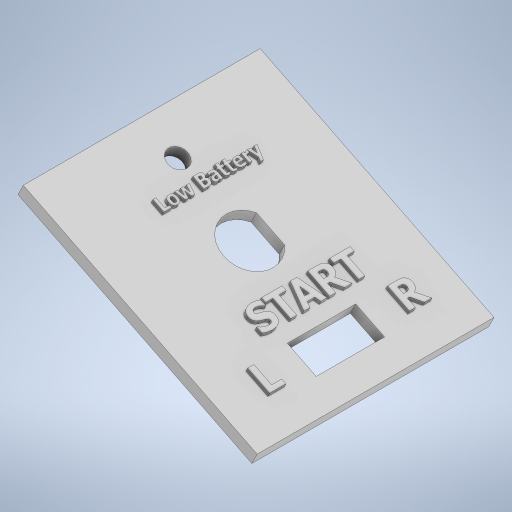
# Autodesk Inventor part: ControlPanel_Top
Saved by Autodesk Inventor 2024.2 (Build 282272000, 272)
## iProperties
Created: 2024-04-16
Part Number: ControlPanel_Top
Material: Generic
Document SubType Name: Modeling
Designer: ringl
Density: 1 g/cm^3
Appearance: Default
Author: ringl
Autodesk Inventor part; units mm, degrees
note: some values were not read from the file. Chosen so that the rebuilt part matches the saved one: direction of "Emboss1".
ref_plane "YZ Plane" through (0, 0, 0) normal (1, 0, 0) x (0, 1, 0)
ref_plane "XZ Plane" through (0, 0, 0) normal (0, 1, 0) x (-1, 0, 0)
ref_plane "XY Plane" through (0, 0, 0) normal (0, 0, 1) x (1, 0, 0)
sketch "Sketch2" plane through (0, 0, 0) normal (0, 0, 1) x (1, 0, 0)
  line L0 (0, 0) -> (1.3327, 2.6877)
  line L1 (1.3327, 2.6877) -> (-36.9173, 21.6547)
  line L2 (-36.9173, 21.6547) -> (-38.25, 18.9669)
  line L3 (-38.25, 18.9669) -> (0, 0)
  line L4 (-38.25, 18.9669) -> (-38.25, 15)
  line L5 (-38.25, 15) -> (-30.25, 15)
  line L6 (-6.5, 3.2231) -> (-6.5, 0)
  line L7 (-6.5, 0) -> (0, 0)
  line L8 (1.3327, 2.6877) -> (21.3327, -7.2296)
  line L9 (21.3327, -7.2296) -> (20, -9.9174)
  line L10 (20, -9.9174) -> (0, 0)
  point P0 (-3.25, 0)
  point P1 (-34.25, 15)
  dimension "d4" = 3
  dimension "d5" = 3
  dimension "d6" = 38.25
  dimension "d8" = 6.5
  dimension "d9" = 8
  dimension "d16" = 15
  dimension "d29" = 20
  constraints: 22 end point, 5 perpendicular, 2 collinear, 2 midpoint, 2 point on line, 2 vertical
  measures "d4" distance of L0.start L0.end
  measures "d5" distance of L1.end L2.end
  measures "d6" horizontal distance of L0.end L1.end
  measures "d8" distance of L6.end L0.start
  measures "d9" distance of L4.end L5.end
  measures "d16" vertical distance of point (-3.25, 0) point (-34.25, 15)
  measures "d29" horizontal distance of L0.end L8.end
extrude "Extrusion1" add sketch "Sketch2" along normal blind 9
sketch "Sketch3" plane through (0, 0, 9) normal (0, 0, 1) x (1, 0, 0)
  line L0 (-38.25, 18.9669) -> (-38.25, 15) projected
  line L1 (-38.25, 15) -> (-30.25, 15) projected
  line L2 (-30.25, 15) -> (-6.5, 3.2231) projected
  line L3 (-6.5, 3.2231) -> (-6.5, 0) projected
  line L4 (-6.5, 0) -> (0, 0) projected
  line L5 (-36.9173, 21.6547) -> (-38.25, 18.9669) projected
  line L6 (-30.25, 15) -> (-38.25, 18.9669)
  line L7 (-6.5, 3.2231) -> (0, 0)
  line L8 (0, 0) -> (20, -9.9174) projected
  line L9 (20, -9.9174) -> (21.3327, -7.2296) projected
  line L10 (21.3327, -7.2296) -> (-36.9173, 21.6547) projected
  constraints: 4 end point
extrude "Extrusion2" add sketch "Sketch3" along normal blind 41 contours L5 L10 L9 L8 L7 L2 L6
sketch "Sketch4" plane through (0, 0, 50) normal (0, 0, 1) x (1, 0, 0)
  line L0 (-38.25, 15) -> (-30.25, 15) projected
  line L1 (-30.25, 15) -> (-38.25, 18.9669) projected
  line L2 (-38.25, 18.9669) -> (-38.25, 15) projected
  line L3 (-38.25, 15) -> (-30.25, 15) projected
  line L4 (-36.9173, 21.6547) -> (-38.25, 18.9669) projected
  line L5 (-38.25, 18.9669) -> (20, -9.9174) projected
  line L6 (0, 0) -> (-6.5, 3.2231) projected
  line L7 (-6.5, 3.2231) -> (-6.5, 0) projected
  line L8 (-6.5, 0) -> (0, 0) projected
  line L9 (20, -9.9174) -> (21.3327, -7.2296) projected
  line L10 (21.3327, -7.2296) -> (-36.9173, 21.6547) projected
  point P0 (-6.5, 3.2231)
extrude "Extrusion3" add sketch "Sketch4" along normal blind 9
sketch "Sketch7" plane through (-36.9173, 21.6547, 59) normal (0.4442495, 0.8959031, 0) x (0.8959031, -0.4442495, 0)
  circle A0 centre (10, 29.5) radius 2.5
  arc A1 (26.1, 34.7) -> (33.9, 34.7) centre (30, 29.5) ccw
  line L0 (50, 21) -> (58, 21)
  line L1 (58, 21) -> (58, 38)
  line L2 (58, 38) -> (50, 38)
  line L3 (50, 38) -> (50, 21)
  line L4 (65.0182, 0) -> (0, 0) projected
  line L5 (26.1, 34.7) -> (33.9, 34.7)
  line L6 (0, 59) -> (0, 0) projected
  point P0 (42.6943, 59)
  point P1 (30, 34.7)
  dimension "d30" = 5
  dimension "d31" = 13
  dimension "d32" = 29.5
  dimension "d33" = 17
  dimension "d34" = 5.2
  dimension "d35" = 10
  dimension "d36" = 20
  dimension "d37" = 8
  dimension "d38" = 8.5
  dimension "d39" = 20
  constraints: 10 end point, 2 centre point, 2 horizontal, 2 parallel, 2 point on circle, 1 horizontal alignment, 1 midpoint, 1 perpendicular
  measures "d30" diameter of A0
  measures "d31" diameter of A1
  measures "d32" distance from line of L4 A0.centre
  measures "d33" distance of L0.end L1.end
  measures "d34" distance of A1.centre point (30, 34.7)
  measures "d35" distance from line of L6 A0.centre
  measures "d36" distance of A0.centre A1.centre
  measures "d37" distance of L1.end L2.end
  measures "d38" distance from line of A1.centre L0
  measures "d39" distance from line of A1.centre L3
extrude "Extrusion5" cut sketch "Sketch7" against normal through all
sketch "Sketch8" plane through (-36.9173, 21.6547, 59) normal (0.4442495, 0.8959031, 0) x (0.8959031, -0.4442495, 0)
  line L0 (50.6129, 9.4648) -> (50.6129, 15.8675) construction
  line L1 (50.6129, 15.8675) -> (57.6973, 15.8675) construction
  line L2 (57.6973, 15.8675) -> (57.6973, 9.4648) construction
  line L3 (57.6973, 9.4648) -> (50.6129, 9.4648) construction
  line L4 (50.3694, 44.5006) -> (50.3694, 50.5681) construction
  line L5 (50.3694, 50.5681) -> (57.1811, 50.5681) construction
  line L6 (57.1811, 50.5681) -> (57.1811, 44.5006) construction
  line L7 (57.1811, 44.5006) -> (50.3694, 44.5006) construction
  line L8 (40.4621, 17.2085) -> (40.4621, 23.6112) construction
  line L9 (40.4621, 23.6112) -> (47.5465, 23.6112) construction
  line L10 (47.5465, 23.6112) -> (47.5465, 17.2085) construction
  line L11 (47.5465, 17.2085) -> (40.4621, 17.2085) construction
  line L12 (19.3245, 18.3628) -> (14.6791, 18.3628) construction
  line L13 (14.6791, 18.3628) -> (14.6791, 42.9569) construction
  line L14 (14.6791, 42.9569) -> (19.3245, 42.9569) construction
  line L15 (19.3245, 42.9569) -> (19.3245, 18.3628) construction
  line L16 (56.7129, 14.1658) -> (56.7129, 10.0975)
  line L17 (56.7129, 10.0975) -> (50.6129, 10.0975)
  line L18 (50.6129, 10.0975) -> (50.6129, 11.6299)
  line L19 (50.6129, 11.6299) -> (55.5512, 11.6299)
  line L20 (55.5512, 11.6299) -> (55.5512, 14.1658)
  line L21 (55.5512, 14.1658) -> (56.7129, 14.1658)
  line L22 (56.4694, 50.7687) -> (56.4694, 48.905)
  line L23 (56.4694, 48.905) -> (54.2301, 47.2095)
  line L24 (54.2301, 47.2095) -> (54.2301, 46.6559)
  line L25 (54.2301, 46.6559) -> (56.4694, 46.6559)
  line L26 (56.4694, 46.6559) -> (56.4694, 45.1333)
  line L27 (56.4694, 45.1333) -> (50.3694, 45.1333)
  line L28 (50.3694, 45.1333) -> (50.3694, 47.5852)
  spline S0 degree 2 poles (50.3694, 47.5852) (50.3694, 48.0943) (50.4979, 48.8457) (50.6956, 49.167) knots 0 0 0 1 2 2 2
  spline S1 degree 2 poles (50.6956, 49.167) (50.9032, 49.4933) (51.5508, 49.8789) (52.0451, 49.8789) knots 0 0 0 1 2 2 2
  spline S2 degree 2 poles (52.0451, 49.8789) (52.7421, 49.8789) (53.6171, 49.2461) (53.8741, 48.7172) knots 0 0 0 1 2 2 2
  line L29 (53.8741, 48.7172) -> (56.4694, 50.7687)
  spline S3 degree 2 poles (52.2379, 48.3069) (52.0056, 48.3069) (51.6744, 48.129) (51.5854, 47.9263) knots 0 0 0 1 2 2 2
  spline S4 degree 2 poles (51.5854, 47.9263) (51.5261, 47.7829) (51.4915, 47.4319) (51.4915, 47.17) knots 0 0 0 1 2 2 2
  line L30 (51.4915, 47.17) -> (51.4915, 46.6559)
  line L31 (51.4915, 46.6559) -> (53.1326, 46.6559)
  line L32 (53.1326, 46.6559) -> (53.1326, 47.0958)
  spline S5 degree 2 poles (53.1326, 47.0958) (53.1326, 47.4122) (53.0536, 47.862) (52.93, 48.0153) knots 0 0 0 1 2 2 2
  spline S6 degree 2 poles (52.93, 48.0153) (52.8113, 48.1636) (52.495, 48.3069) (52.2379, 48.3069) knots 0 0 0 1 2 2 2
  spline S7 degree 2 poles (46.7796, 19.7246) (46.7796, 19.0227) (46.5077, 17.9648) (46.31, 17.51) knots 0 0 0 1 2 2 2
  line L33 (46.31, 17.51) -> (44.8567, 17.51)
  line L34 (44.8567, 17.51) -> (44.8567, 17.6484)
  spline S8 degree 2 poles (44.8567, 17.6484) (45.2472, 18.1081) (45.6674, 19.2105) (45.6674, 19.7295) knots 0 0 0 1 2 2 2
  spline S9 degree 2 poles (45.6674, 19.7295) (45.6674, 19.863) (45.6081, 20.2931) (45.5487, 20.4216) knots 0 0 0 1 2 2 2
  spline S10 degree 2 poles (45.5487, 20.4216) (45.4795, 20.5798) (45.2274, 20.8022) (45.0248, 20.8022) knots 0 0 0 1 2 2 2
  spline S11 degree 2 poles (45.0248, 20.8022) (44.7924, 20.8022) (44.5057, 20.4414) (44.4415, 20.1942) knots 0 0 0 1 2 2 2
  spline S12 degree 2 poles (44.4415, 20.1942) (44.3574, 19.8828) (44.2141, 19.1759) (44.1053, 18.8645) knots 0 0 0 1 2 2 2
  spline S13 degree 2 poles (44.1053, 18.8645) (43.8581, 18.1576) (43.0128, 17.5446) (42.3801, 17.5446) knots 0 0 0 1 2 2 2
  spline S14 degree 2 poles (42.3801, 17.5446) (41.5249, 17.5446) (40.4621, 18.993) (40.4621, 20.0805) knots 0 0 0 1 2 2 2
  spline S15 degree 2 poles (40.4621, 20.0805) (40.4621, 20.6243) (40.6846, 21.7019) (40.8724, 22.127) knots 0 0 0 1 2 2 2
  line L35 (40.8724, 22.127) -> (42.2664, 22.127)
  line L36 (42.2664, 22.127) -> (42.2664, 21.9936)
  spline S16 degree 2 poles (42.2664, 21.9936) (41.9748, 21.6525) (41.5744, 20.6737) (41.5744, 20.1596) knots 0 0 0 1 2 2 2
  spline S17 degree 2 poles (41.5744, 20.1596) (41.5744, 19.9569) (41.6337, 19.6406) (41.7128, 19.4626) knots 0 0 0 1 2 2 2
  spline S18 degree 2 poles (41.7128, 19.4626) (41.777, 19.3193) (42.0341, 19.1116) (42.1923, 19.1116) knots 0 0 0 1 2 2 2
  spline S19 degree 2 poles (42.1923, 19.1116) (42.4295, 19.1116) (42.7014, 19.4428) (42.8102, 19.9174) knots 0 0 0 1 2 2 2
  spline S20 degree 2 poles (42.8102, 19.9174) (42.8794, 20.2239) (43.0128, 20.7923) (43.1265, 21.1186) knots 0 0 0 1 2 2 2
  spline S21 degree 2 poles (43.1265, 21.1186) (43.3589, 21.7513) (44.13, 22.3693) (44.7628, 22.3693) knots 0 0 0 1 2 2 2
  spline S22 degree 2 poles (44.7628, 22.3693) (45.6723, 22.3693) (46.7796, 20.9406) (46.7796, 19.7246) knots 0 0 0 1 2 2 2
  line L37 (46.6709, 24.3268) -> (41.7325, 24.3268)
  line L38 (41.7325, 24.3268) -> (41.7325, 22.5225)
  line L39 (41.7325, 22.5225) -> (40.5709, 22.5225)
  line L40 (40.5709, 22.5225) -> (40.5709, 27.6635)
  line L41 (40.5709, 27.6635) -> (41.7325, 27.6635)
  line L42 (41.7325, 27.6635) -> (41.7325, 25.8592)
  line L43 (41.7325, 25.8592) -> (46.6709, 25.8592)
  line L44 (46.6709, 25.8592) -> (46.6709, 24.3268)
  line L45 (46.6709, 27.6338) -> (40.5709, 29.6952)
  line L46 (40.5709, 29.6952) -> (40.5709, 31.366)
  line L47 (40.5709, 31.366) -> (46.6709, 33.4274)
  line L48 (46.6709, 33.4274) -> (46.6709, 31.8505)
  line L49 (46.6709, 31.8505) -> (45.4252, 31.4698)
  line L50 (45.4252, 31.4698) -> (45.4252, 29.5518)
  line L51 (45.4252, 29.5518) -> (46.6709, 29.1663)
  line L52 (46.6709, 29.1663) -> (46.6709, 27.6338)
  line L53 (44.3179, 31.1337) -> (42.301, 30.5108)
  line L54 (42.301, 30.5108) -> (44.3179, 29.883)
  line L55 (44.3179, 29.883) -> (44.3179, 31.1337)
  line L56 (46.6709, 39.6707) -> (46.6709, 37.8071)
  line L57 (46.6709, 37.8071) -> (44.4316, 36.1116)
  line L58 (44.4316, 36.1116) -> (44.4316, 35.5579)
  line L59 (44.4316, 35.5579) -> (46.6709, 35.5579)
  line L60 (46.6709, 35.5579) -> (46.6709, 34.0354)
  line L61 (46.6709, 34.0354) -> (40.5709, 34.0354)
  line L62 (40.5709, 34.0354) -> (40.5709, 36.4872)
  spline S23 degree 2 poles (40.5709, 36.4872) (40.5709, 36.9964) (40.6994, 37.7478) (40.8971, 38.0691) knots 0 0 0 1 2 2 2
  spline S24 degree 2 poles (40.8971, 38.0691) (41.1047, 38.3953) (41.7523, 38.7809) (42.2466, 38.7809) knots 0 0 0 1 2 2 2
  spline S25 degree 2 poles (42.2466, 38.7809) (42.9436, 38.7809) (43.8186, 38.1482) (44.0757, 37.6193) knots 0 0 0 1 2 2 2
  line L63 (44.0757, 37.6193) -> (46.6709, 39.6707)
  spline S26 degree 2 poles (42.4394, 37.209) (42.2071, 37.209) (41.8759, 37.031) (41.7869, 36.8283) knots 0 0 0 1 2 2 2
  spline S27 degree 2 poles (41.7869, 36.8283) (41.7276, 36.685) (41.693, 36.334) (41.693, 36.072) knots 0 0 0 1 2 2 2
  line L64 (41.693, 36.072) -> (41.693, 35.5579)
  line L65 (41.693, 35.5579) -> (43.3342, 35.5579)
  line L66 (43.3342, 35.5579) -> (43.3342, 35.9979)
  spline S28 degree 2 poles (43.3342, 35.9979) (43.3342, 36.3142) (43.2551, 36.7641) (43.1315, 36.9173) knots 0 0 0 1 2 2 2
  spline S29 degree 2 poles (43.1315, 36.9173) (43.0128, 37.0656) (42.6965, 37.209) (42.4394, 37.209) knots 0 0 0 1 2 2 2
  line L67 (46.6709, 41.297) -> (41.7325, 41.297)
  line L68 (41.7325, 41.297) -> (41.7325, 39.4928)
  line L69 (41.7325, 39.4928) -> (40.5709, 39.4928)
  line L70 (40.5709, 39.4928) -> (40.5709, 44.6338)
  line L71 (40.5709, 44.6338) -> (41.7325, 44.6338)
  line L72 (41.7325, 44.6338) -> (41.7325, 42.8295)
  line L73 (41.7325, 42.8295) -> (46.6709, 42.8295)
  line L74 (46.6709, 42.8295) -> (46.6709, 41.297)
  line L75 (17.7291, 20.7134) -> (17.7291, 18.6792)
  line L76 (17.7291, 18.6792) -> (14.6791, 18.6792)
  line L77 (14.6791, 18.6792) -> (14.6791, 19.4454)
  line L78 (14.6791, 19.4454) -> (17.1483, 19.4454)
  line L79 (17.1483, 19.4454) -> (17.1483, 20.7134)
  line L80 (17.1483, 20.7134) -> (17.7291, 20.7134)
  spline S30 degree 2 poles (16.5798, 23.2443) (17.1483, 23.2443) (17.8008, 22.6239) (17.8008, 22.0579) knots 0 0 0 1 2 2 2
  spline S31 degree 2 poles (17.8008, 22.0579) (17.8008, 21.4944) (17.1483, 20.8691) (16.5798, 20.8691) knots 0 0 0 1 2 2 2
  spline S32 degree 2 poles (16.5798, 20.8691) (16.0064, 20.8691) (15.3563, 21.4944) (15.3563, 22.0579) knots 0 0 0 1 2 2 2
  spline S33 degree 2 poles (15.3563, 22.0579) (15.3563, 22.6215) (16.0088, 23.2443) (16.5798, 23.2443) knots 0 0 0 1 2 2 2
  spline S34 degree 2 poles (16.5847, 22.5102) (16.3796, 22.5102) (16.1052, 22.4435) (16.0237, 22.3842) knots 0 0 0 1 2 2 2
  spline S35 degree 2 poles (16.0237, 22.3842) (15.9372, 22.3199) (15.8704, 22.1593) (15.8704, 22.0579) knots 0 0 0 1 2 2 2
  spline S36 degree 2 poles (15.8704, 22.0579) (15.8704, 21.9591) (15.9298, 21.8033) (16.0138, 21.7391) knots 0 0 0 1 2 2 2
  spline S37 degree 2 poles (16.0138, 21.7391) (16.0929, 21.6773) (16.3722, 21.6031) (16.5847, 21.6031) knots 0 0 0 1 2 2 2
  spline S38 degree 2 poles (16.5847, 21.6031) (16.7948, 21.6031) (17.0543, 21.6724) (17.1334, 21.7292) knots 0 0 0 1 2 2 2
  spline S39 degree 2 poles (17.1334, 21.7292) (17.2125, 21.786) (17.2867, 21.9591) (17.2867, 22.0629) knots 0 0 0 1 2 2 2
  spline S40 degree 2 poles (17.2867, 22.0629) (17.2867, 22.1494) (17.2125, 22.3273) (17.1384, 22.3817) knots 0 0 0 1 2 2 2
  spline S41 degree 2 poles (17.1384, 22.3817) (17.0519, 22.4435) (16.8022, 22.5102) (16.5847, 22.5102) knots 0 0 0 1 2 2 2
  line L81 (15.428, 27.0531) -> (17.7291, 26.3808)
  line L82 (17.7291, 26.3808) -> (17.7291, 25.6196)
  line L83 (17.7291, 25.6196) -> (16.2412, 25.2142)
  line L84 (16.2412, 25.2142) -> (17.7291, 24.8089)
  line L85 (17.7291, 24.8089) -> (17.7291, 24.0476)
  line L86 (17.7291, 24.0476) -> (15.428, 23.3803)
  line L87 (15.428, 23.3803) -> (15.428, 24.1341)
  line L88 (15.428, 24.1341) -> (16.9505, 24.4875)
  line L89 (16.9505, 24.4875) -> (15.428, 24.9226)
  line L90 (15.428, 24.9226) -> (15.428, 25.5578)
  line L91 (15.428, 25.5578) -> (16.9505, 25.9681)
  line L92 (16.9505, 25.9681) -> (15.428, 26.3166)
  line L93 (15.428, 26.3166) -> (15.428, 27.0531)
  spline S42 degree 2 poles (16.7948, 31.0646) (17.0222, 31.0646) (17.3658, 30.8916) (17.4795, 30.7482) knots 0 0 0 1 2 2 2
  spline S43 degree 2 poles (17.4795, 30.7482) (17.6154, 30.5752) (17.7291, 30.1649) (17.7291, 29.8461) knots 0 0 0 1 2 2 2
  line L94 (17.7291, 29.8461) -> (17.7291, 28.6275)
  line L95 (17.7291, 28.6275) -> (14.6791, 28.6275)
  line L96 (14.6791, 28.6275) -> (14.6791, 29.7027)
  spline S44 degree 2 poles (14.6791, 29.7027) (14.6791, 30.0388) (14.731, 30.3849) (14.8126, 30.5356) knots 0 0 0 1 2 2 2
  spline S45 degree 2 poles (14.8126, 30.5356) (14.8991, 30.7012) (15.1957, 30.8619) (15.3885, 30.8619) knots 0 0 0 1 2 2 2
  spline S46 degree 2 poles (15.3885, 30.8619) (15.6109, 30.8619) (15.9594, 30.6395) (16.041, 30.4417) knots 0 0 0 1 2 2 2
  line L97 (16.041, 30.4417) -> (16.0558, 30.4417)
  spline S47 degree 2 poles (16.0558, 30.4417) (16.1151, 30.726) (16.4834, 31.0646) (16.7948, 31.0646) knots 0 0 0 1 2 2 2
  spline S48 degree 2 poles (16.7825, 30.2736) (16.6391, 30.2736) (16.4785, 30.16) (16.4364, 30.0463) knots 0 0 0 1 2 2 2
  spline S49 degree 2 poles (16.4364, 30.0463) (16.4092, 29.9771) (16.4043, 29.7324) (16.4043, 29.5297) knots 0 0 0 1 2 2 2
  line L98 (16.4043, 29.5297) -> (16.4043, 29.3888)
  line L99 (16.4043, 29.3888) -> (17.173, 29.3888)
  line L100 (17.173, 29.3888) -> (17.173, 29.4308)
  spline S50 degree 2 poles (17.173, 29.4308) (17.173, 29.7274) (17.1656, 29.9548) (17.1137, 30.0734) knots 0 0 0 1 2 2 2
  spline S51 degree 2 poles (17.1137, 30.0734) (17.0667, 30.1773) (16.8937, 30.2736) (16.7825, 30.2736) knots 0 0 0 1 2 2 2
  spline S52 degree 2 poles (15.5392, 30.0833) (15.4651, 30.0833) (15.3094, 30.0067) (15.2748, 29.9276) knots 0 0 0 1 2 2 2
  spline S53 degree 2 poles (15.2748, 29.9276) (15.2402, 29.8535) (15.2352, 29.6459) (15.2352, 29.4407) knots 0 0 0 1 2 2 2
  line L101 (15.2352, 29.4407) -> (15.2352, 29.3888)
  line L102 (15.2352, 29.3888) -> (15.8828, 29.3888)
  line L103 (15.8828, 29.3888) -> (15.8828, 29.4852)
  spline S54 degree 2 poles (15.8828, 29.4852) (15.8828, 29.6805) (15.8754, 29.8386) (15.8358, 29.9227) knots 0 0 0 1 2 2 2
  spline S55 degree 2 poles (15.8358, 29.9227) (15.7913, 30.0141) (15.6406, 30.0833) (15.5392, 30.0833) knots 0 0 0 1 2 2 2
  spline S56 degree 2 poles (17.4844, 32.7305) (17.5462, 32.6563) (17.6451, 32.5401) (17.6945, 32.4413) knots 0 0 0 1 2 2 2
  spline S57 degree 2 poles (17.6945, 32.4413) (17.7415, 32.3449) (17.7909, 32.162) (17.7909, 31.9989) knots 0 0 0 1 2 2 2
  spline S58 degree 2 poles (17.7909, 31.9989) (17.7909, 31.6924) (17.3806, 31.2895) (17.0692, 31.2895) knots 0 0 0 1 2 2 2
  spline S59 degree 2 poles (17.0692, 31.2895) (16.8146, 31.2895) (16.4982, 31.4946) (16.4068, 31.6874) knots 0 0 0 1 2 2 2
  spline S60 degree 2 poles (16.4068, 31.6874) (16.3129, 31.8827) (16.2387, 32.424) (16.2189, 32.7354) knots 0 0 0 1 2 2 2
  line L104 (16.2189, 32.7354) -> (16.2066, 32.7354)
  spline S61 degree 2 poles (16.2066, 32.7354) (16.0163, 32.7354) (15.8704, 32.4536) (15.8704, 32.1719) knots 0 0 0 1 2 2 2
  spline S62 degree 2 poles (15.8704, 32.1719) (15.8704, 32.0458) (15.9619, 31.7047) (16.0336, 31.5441) knots 0 0 0 1 2 2 2
  line L105 (16.0336, 31.5441) -> (16.0336, 31.4823)
  line L106 (16.0336, 31.4823) -> (15.4774, 31.4823)
  spline S63 degree 2 poles (15.4774, 31.4823) (15.4478, 31.5886) (15.3637, 32.0631) (15.3637, 32.3053) knots 0 0 0 1 2 2 2
  spline S64 degree 2 poles (15.3637, 32.3053) (15.3637, 32.8985) (15.7592, 33.4423) (16.1646, 33.4423) knots 0 0 0 1 2 2 2
  line L107 (16.1646, 33.4423) -> (17.7291, 33.4423)
  line L108 (17.7291, 33.4423) -> (17.7291, 32.7305)
  line L109 (17.7291, 32.7305) -> (17.4844, 32.7305)
  line L110 (17.1285, 32.7305) -> (16.6515, 32.7305)
  spline S65 degree 2 poles (16.6515, 32.7305) (16.6688, 32.5476) (16.696, 32.3226) (16.7355, 32.2139) knots 0 0 0 1 2 2 2
  spline S66 degree 2 poles (16.7355, 32.2139) (16.7676, 32.1175) (16.9011, 32.0137) (17.0099, 32.0137) knots 0 0 0 1 2 2 2
  spline S67 degree 2 poles (17.0099, 32.0137) (17.1705, 32.0137) (17.2916, 32.1892) (17.2916, 32.3597) knots 0 0 0 1 2 2 2
  spline S68 degree 2 poles (17.2916, 32.3597) (17.2916, 32.4536) (17.2051, 32.6514) (17.1285, 32.7305) knots 0 0 0 1 2 2 2
  spline S69 degree 2 poles (17.7736, 34.8536) (17.7736, 34.4161) (17.4127, 34.0157) (17.0024, 34.0157) knots 0 0 0 1 2 2 2
  line L111 (17.0024, 34.0157) -> (15.9273, 34.0157)
  line L112 (15.9273, 34.0157) -> (15.9273, 33.7414)
  line L113 (15.9273, 33.7414) -> (15.428, 33.7414)
  line L114 (15.428, 33.7414) -> (15.428, 34.0157)
  line L115 (15.428, 34.0157) -> (14.7706, 34.0157)
  line L116 (14.7706, 34.0157) -> (14.7706, 34.7325)
  line L117 (14.7706, 34.7325) -> (15.428, 34.7325)
  line L118 (15.428, 34.7325) -> (15.428, 35.4245)
  line L119 (15.428, 35.4245) -> (15.9273, 35.4245)
  line L120 (15.9273, 35.4245) -> (15.9273, 34.7325)
  line L121 (15.9273, 34.7325) -> (16.7454, 34.7325)
  spline S70 degree 2 poles (16.7454, 34.7325) (16.8665, 34.7325) (17.0469, 34.7374) (17.1186, 34.7671) knots 0 0 0 1 2 2 2
  spline S71 degree 2 poles (17.1186, 34.7671) (17.1903, 34.7967) (17.2743, 34.9426) (17.2743, 35.081) knots 0 0 0 1 2 2 2
  spline S72 degree 2 poles (17.2743, 35.081) (17.2743, 35.1403) (17.2249, 35.3257) (17.2051, 35.3628) knots 0 0 0 1 2 2 2
  line L122 (17.2051, 35.3628) -> (17.2051, 35.4245)
  line L123 (17.2051, 35.4245) -> (17.7093, 35.4245)
  spline S73 degree 2 poles (17.7093, 35.4245) (17.739, 35.3084) (17.7736, 35.0464) (17.7736, 34.8536) knots 0 0 0 1 2 2 2
  spline S74 degree 2 poles (17.7736, 36.5961) (17.7736, 36.1586) (17.4127, 35.7582) (17.0024, 35.7582) knots 0 0 0 1 2 2 2
  line L124 (17.0024, 35.7582) -> (15.9273, 35.7582)
  line L125 (15.9273, 35.7582) -> (15.9273, 35.4839)
  line L126 (15.9273, 35.4839) -> (15.428, 35.4839)
  line L127 (15.428, 35.4839) -> (15.428, 35.7582)
  line L128 (15.428, 35.7582) -> (14.7706, 35.7582)
  line L129 (14.7706, 35.7582) -> (14.7706, 36.475)
  line L130 (14.7706, 36.475) -> (15.428, 36.475)
  line L131 (15.428, 36.475) -> (15.428, 37.167)
  line L132 (15.428, 37.167) -> (15.9273, 37.167)
  line L133 (15.9273, 37.167) -> (15.9273, 36.475)
  line L134 (15.9273, 36.475) -> (16.7454, 36.475)
  spline S75 degree 2 poles (16.7454, 36.475) (16.8665, 36.475) (17.0469, 36.4799) (17.1186, 36.5096) knots 0 0 0 1 2 2 2
  spline S76 degree 2 poles (17.1186, 36.5096) (17.1903, 36.5392) (17.2743, 36.6851) (17.2743, 36.8235) knots 0 0 0 1 2 2 2
  spline S77 degree 2 poles (17.2743, 36.8235) (17.2743, 36.8828) (17.2249, 37.0682) (17.2051, 37.1053) knots 0 0 0 1 2 2 2
  line L135 (17.2051, 37.1053) -> (17.2051, 37.167)
  line L136 (17.2051, 37.167) -> (17.7093, 37.167)
  spline S78 degree 2 poles (17.7093, 37.167) (17.739, 37.0509) (17.7736, 36.7889) (17.7736, 36.5961) knots 0 0 0 1 2 2 2
  spline S79 degree 2 poles (17.7909, 38.6377) (17.7909, 37.9852) (17.168, 37.2906) (16.5922, 37.2906) knots 0 0 0 1 2 2 2
  spline S80 degree 2 poles (16.5922, 37.2906) (16.0286, 37.2906) (15.3563, 37.9382) (15.3563, 38.5215) knots 0 0 0 1 2 2 2
  spline S81 degree 2 poles (15.3563, 38.5215) (15.3563, 39.048) (15.9273, 39.5818) (16.4562, 39.5818) knots 0 0 0 1 2 2 2
  line L137 (16.4562, 39.5818) -> (16.7157, 39.5818)
  line L138 (16.7157, 39.5818) -> (16.7157, 38.0074)
  spline S82 degree 2 poles (16.7157, 38.0074) (16.8764, 38.0173) (17.0889, 38.1335) (17.1532, 38.2274) knots 0 0 0 1 2 2 2
  spline S83 degree 2 poles (17.1532, 38.2274) (17.2175, 38.3188) (17.2719, 38.566) (17.2719, 38.7118) knots 0 0 0 1 2 2 2
  spline S84 degree 2 poles (17.2719, 38.7118) (17.2719, 38.8354) (17.2175, 39.0776) (17.1705, 39.179) knots 0 0 0 1 2 2 2
  spline S85 degree 2 poles (17.1705, 39.179) (17.1334, 39.2679) (17.042, 39.4162) (17.0074, 39.4632) knots 0 0 0 1 2 2 2
  line L139 (17.0074, 39.4632) -> (17.0074, 39.5398)
  line L140 (17.0074, 39.5398) -> (17.6006, 39.5398)
  spline S86 degree 2 poles (17.6006, 39.5398) (17.6352, 39.4508) (17.6945, 39.3075) (17.7242, 39.179) knots 0 0 0 1 2 2 2
  spline S87 degree 2 poles (17.7242, 39.179) (17.7563, 39.0628) (17.7909, 38.8156) (17.7909, 38.6377) knots 0 0 0 1 2 2 2
  spline S88 degree 2 poles (16.2832, 38.8749) (16.0558, 38.87) (15.8161, 38.6698) (15.8161, 38.4647) knots 0 0 0 1 2 2 2
  spline S89 degree 2 poles (15.8161, 38.4647) (15.8161, 38.2546) (16.0682, 38.0173) (16.2832, 38.0049) knots 0 0 0 1 2 2 2
  line L141 (16.2832, 38.0049) -> (16.2832, 38.8749)
  line L142 (16.1077, 41.4949) -> (16.1077, 41.4356)
  spline S90 degree 2 poles (16.1077, 41.4356) (16.0929, 41.3935) (16.0781, 41.2378) (16.0781, 41.1439) knots 0 0 0 1 2 2 2
  spline S91 degree 2 poles (16.0781, 41.1439) (16.0781, 41.0327) (16.1448, 40.7831) (16.1893, 40.6669) knots 0 0 0 1 2 2 2
  line L143 (16.1893, 40.6669) -> (17.7291, 40.6669)
  line L144 (17.7291, 40.6669) -> (17.7291, 39.9501)
  line L145 (17.7291, 39.9501) -> (15.428, 39.9501)
  line L146 (15.428, 39.9501) -> (15.428, 40.6669)
  line L147 (15.428, 40.6669) -> (15.7592, 40.6669)
  spline S92 degree 2 poles (15.7592, 40.6669) (15.7147, 40.7163) (15.5763, 40.8893) (15.5343, 40.961) knots 0 0 0 1 2 2 2
  spline S93 degree 2 poles (15.5343, 40.961) (15.4873, 41.0401) (15.4206, 41.2477) (15.4206, 41.3392) knots 0 0 0 1 2 2 2
  spline S94 degree 2 poles (15.4206, 41.3392) (15.4206, 41.3738) (15.4255, 41.4603) (15.428, 41.4949) knots 0 0 0 1 2 2 2
  line L148 (15.428, 41.4949) -> (16.1077, 41.4949)
  line L149 (15.428, 43.9146) -> (18.5719, 42.7554)
  line L150 (18.5719, 42.7554) -> (18.5719, 41.9843)
  line L151 (18.5719, 41.9843) -> (17.6723, 42.3328)
  line L152 (17.6723, 42.3328) -> (15.428, 41.4899)
  line L153 (15.428, 41.4899) -> (15.428, 42.2413)
  line L154 (15.428, 42.2413) -> (16.8714, 42.7258)
  line L155 (16.8714, 42.7258) -> (15.428, 43.1781)
  line L156 (15.428, 43.1781) -> (15.428, 43.9146)
  point P0 (42.6943, 59)
  constraints: 8 other
emboss "Emboss1" sketch "Sketch8" operation add depth 1 direction (-0.4442495, -0.8959031, 0)
sketch "Sketch9" plane through (-6.5, 0, 50) normal (0, -1, 0) x (1, 0, 0)
  circle A0 centre (3.25, 4) radius 1.5
  circle A1 centre (3.25, -45) radius 1.5
  line L0 (0, 0) -> (0, 9) projected
  line L1 (0, -50) -> (0, -41) projected
  line L2 (0, 0) -> (6.5, 0) projected
  point P0 (6.5, -50)
  point P1 (3.25, 0)
  dimension "d44" = 49
  dimension "d45" = 3
  dimension "d46" = 3
  dimension "d47" = 3.25
  dimension "d48" = 3.25
  dimension "d49" = 4
  constraints: 2 centre point, 1 midpoint
  measures "d44" distance of A0.centre A1.centre
  measures "d45" diameter of A0
  measures "d46" diameter of A1
  measures "d47" distance from line of L0 A0.centre
  measures "d48" distance from line of L1 A1.centre
  measures "d49" distance of A0.centre point (3.25, 0)
extrude "Extrusion6" add sketch "Sketch9" along normal blind 2.5
sketch "Sketch10" plane through (-38.25, 15, 0) normal (0, -1, 0) x (1, 0, 0)
  circle A0 centre (4, 4) radius 1.5
  circle A1 centre (4, 55) radius 1.5
  line L0 (0, 0) -> (8, 0) projected
  line L1 (0, 50) -> (0, 59) projected
  point P0 (38.25, 0)
  dimension "d52" = 3
  dimension "d53" = 3
  dimension "d54" = 51
  dimension "d55" = 4
  dimension "d56" = 4
  constraints: 2 centre point, 1 vertical alignment
  measures "d52" diameter of A0
  measures "d53" diameter of A1
  measures "d54" distance of A0.centre A1.centre
  measures "d55" distance from line of L0 A0.centre
  measures "d56" distance from line of L1 A1.centre
extrude "Extrusion7" add sketch "Sketch10" along normal blind 2.5
sketch "Sketch11" plane through (21.3327, -7.2296, 59) normal (0.8959031, -0.4442495, 0) x (0, 0, -1)
  line L0 (9, -3) -> (0, -3) projected
  line L1 (0, -3) -> (-12.6421, -15.6421)
  line L2 (-12.6421, -15.6421) -> (-14.1421, -14.1421)
  line L3 (59, 0) -> (0, 0) projected
  line L4 (-14.1421, -14.1421) -> (0, 0)
  line L5 (59, 0) -> (73.1421, -14.1421)
  line L6 (73.1421, -14.1421) -> (71.6421, -15.6421)
  line L7 (71.6421, -15.6421) -> (59, -3)
  line L8 (59, -3) -> (50, -3) projected
  line L9 (59, -3) -> (59, 0)
  line L10 (0, 0) -> (0, -3)
  point P0 (59, -3)
  dimension "d59" = 135
  dimension "d60" = 20
  dimension "d61" = 135
  dimension "d62" = 20
  constraints: 16 end point, 6 perpendicular, 1 coincident
  measures "d59" angle of L0 L1
  measures "d60" distance of L2.end L3.end
  measures "d61" angle of L8 L7
  measures "d62" distance of L3.start L5.end
extrude "Extrusion8" [suppressed]
sketch "Sketch12" plane through (0, 0, 59) normal (0, 0, 1) x (1, 0, 0)
  line L0 (-38.25, 18.9669) -> (-30.25, 15) projected
  line L1 (-38.25, 18.9669) -> (20, -9.9174)
  line L2 (20, -9.9174) -> (-38.25, -9.9174)
  line L3 (-38.25, 18.9669) -> (-38.25, 15) projected
  line L4 (-38.25, -9.9174) -> (-38.25, 18.9669)
  point P0 (0, 0)
  constraints: 6 end point, 2 collinear, 1 coincident, 1 horizontal
extrude "Extrusion9" cut sketch "Sketch12" against normal through all
body "Solid1"
